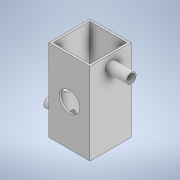
# Autodesk Inventor part: Part2
Saved by Autodesk Inventor 2022 (Build 260153070, 153G)
## iProperties
Created: 2021-07-14
Part Number: Part2
Material: Generic
Document SubType Name: Modeling
Designer: Eakawit_kor
Density: 1 g/cm^3
Appearance: Default
Author: Eakawit_kor
Autodesk Inventor part; units mm, degrees
ref_plane "YZ Plane" through (0, 0, 0) normal (1, 0, 0) x (0, 1, 0)
ref_plane "XZ Plane" through (0, 0, 0) normal (0, 1, 0) x (-1, 0, 0)
ref_plane "XY Plane" through (0, 0, 0) normal (0, 0, 1) x (1, 0, 0)
sketch "Sketch1" plane through (0, 0, 0) normal (0, 0, 1) x (1, 0, 0)
  line L0 (0, 0) -> (20, 0)
  line L1 (20, 0) -> (20, 40)
  line L2 (20, 40) -> (0, 40)
  line L3 (0, 40) -> (0, 0)
  dimension "d2" = 20
  dimension "d3" = 40
  constraints: 8 end point, 2 parallel, 1 horizontal, 1 perpendicular
  measures "d2" distance of L1.end L2.end
  measures "d3" distance of L2.end L0.start
extrude "Extrusion1" add sketch "Sketch1" along normal blind 20
sketch "Sketch2" plane through (0, 0, 0) normal (-1, 0, 0) x (0, 0, 1)
  circle A0 centre (10, 5) radius 2.5
  line L0 (0, 0) -> (20, 0) projected
  line L1 (0, 40) -> (0, 0) projected
  dimension "d6" = 5
  dimension "d7" = 5
  dimension "d8" = 10
  constraints: 1 centre point
  measures "d6" diameter of A0
  measures "d7" distance from line of L0 A0.centre
  measures "d8" distance from line of L1 A0.centre
extrude "Extrusion2" add sketch "Sketch2" along normal blind 10
sketch "Sketch3" plane through (20, 0, 0) normal (1, 0, 0) x (0, 0, -1)
  circle A0 centre (-10, 35) radius 2.5
  line L0 (0, 40) -> (-20, 40) projected
  line L1 (0, 0) -> (0, 40) projected
  dimension "d11" = 5
  dimension "d12" = 5
  dimension "d13" = 10
  constraints: 1 centre point
  measures "d11" diameter of A0
  measures "d12" distance from line of L0 A0.centre
  measures "d13" distance from line of L1 A0.centre
extrude "Extrusion3" add sketch "Sketch3" along normal blind 10
sketch "Sketch4" plane through (0, 0, 20) normal (0, 0, 1) x (1, 0, 0)
  circle A0 centre (10, 20) radius 5
  line L0 (0, 0) -> (20, 0) projected
  line L1 (0, 40) -> (0, 0) projected
  dimension "d16" = 10
  dimension "d17" = 20
  dimension "d18" = 10
  constraints: 1 centre point
  measures "d16" diameter of A0
  measures "d17" distance from line of L0 A0.centre
  measures "d18" distance from line of L1 A0.centre
extrude "Extrusion4" cut sketch "Sketch4" against normal blind 20
sketch "Sketch6" plane through (0, 0, 0) normal (-1, 0, 0) x (0, 0, 1)
  circle A0 centre (10, 20) radius 5
  line L0 (0, 40) -> (0, 0) projected
  line L1 (0, 0) -> (20, 0) projected
  dimension "d27" = 10
  dimension "d28" = 10
  dimension "d29" = 20
  constraints: 1 centre point
  measures "d27" diameter of A0
  measures "d28" distance from line of L0 A0.centre
  measures "d29" distance from line of L1 A0.centre
sketch "Sketch9" plane through (0, 40, 0) normal (0, 1, 0) x (1, 0, 0)
  line L0 (1, -1) -> (19, -1)
  line L1 (19, -1) -> (19, -19)
  line L2 (19, -19) -> (1, -19)
  line L3 (1, -19) -> (1, -1)
  line L4 (0, 0) -> (0, -20) projected
  line L5 (20, 0) -> (0, 0) projected
  line L6 (20, 0) -> (20, -20) projected
  line L7 (20, -20) -> (0, -20) projected
  dimension "d32" = 1
  dimension "d33" = 1
  dimension "d34" = 1
  dimension "d35" = 1
  constraints: 8 end point, 2 parallel, 1 horizontal, 1 perpendicular
  measures "d32" distance between parallel lines of L4 L3
  measures "d33" distance between parallel lines of L5 L0
  measures "d34" distance between parallel lines of L6 L1
  measures "d35" distance between parallel lines of L7 L2
extrude "Extrusion7" cut sketch "Sketch9" against normal blind 39 contours L0 L1 L2 L3
extrude "Extrusion8" cut sketch "Sketch6" against normal up to surface (1 mm away)
sketch "Sketch10" plane through (-10, 5, 10) normal (-1, 0, 0) x (0, 0, 1)
  circle A0 centre (0, 0) radius 2
  circle A1 centre (0, 0) radius 2.5 projected
  point P0 (-10, -5)
  dimension "d40" = 0.5
  constraints: 1 centre point, 1 concentric
  measures "d40" radial gap between concentric circles of A1 A0
extrude "Extrusion9" cut sketch "Sketch10" against normal blind 11 contours A0
sketch "Sketch11" plane through (30, 35, 10) normal (1, 0, 0) x (0, 0, -1)
  circle A0 centre (0, 0) radius 2
  circle A1 centre (0, 0) radius 2.5 projected
  point P0 (10, -35)
  dimension "d43" = 0.5
  constraints: 1 centre point, 1 concentric
  measures "d43" radial gap between concentric circles of A1 A0
extrude "Extrusion10" cut sketch "Sketch11" against normal blind 11 contours A0
body "Solid1"
